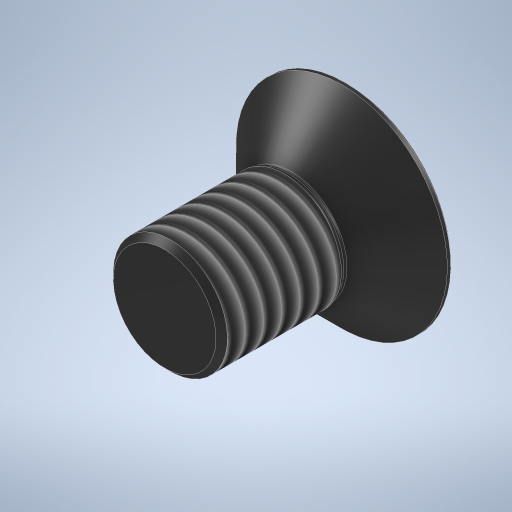
# Autodesk Inventor part: FSCM5x8
Saved by Autodesk Inventor 2024 (Build 280153000, 153)
## iProperties
Created: 2024-09-05
Part Number: FSCM5x8
Material: Stainless Steel
Document SubType Name: Modeling
Designer: Ishaan
Density: 8 g/cm^3
Appearance: Iron Gray
Author: Ishaan
Autodesk Inventor part; units mm, degrees
ref_plane "YZ Plane" through (0, 0, 0) normal (1, 0, 0) x (0, 1, 0)
ref_plane "XZ Plane" through (0, 0, 0) normal (0, 1, 0) x (-1, 0, 0)
ref_plane "XY Plane" through (0, 0, 0) normal (0, 0, 1) x (1, 0, 0)
sketch "Sketch3" plane through (0, 0, 0) normal (1, 0, 0) x (0, 1, 0)
  line L0 (0, 0) -> (0, 8)
  line L1 (0, 8) -> (2.5, 8)
  line L2 (2.5, 8) -> (2.5, 2.6578)
  line L3 (2.5, 2.6578) -> (2.4293, 2.5871)
  line L4 (4.625, 0) -> (0, 0)
  line L5 (2.4293, 2.4457) -> (4.625, 0.25)
  line L6 (4.625, 0.25) -> (4.625, 0)
  arc A0 (2.4293, 2.5871) -> (2.4293, 2.4457) centre (2.5, 2.5164) ccw
  dimension "d37" = 4.625
  dimension "d38" = 2.5
  dimension "d39" = 8
  dimension "d40" = 0.25
  dimension "d41" = 45
  dimension "d42" = 0.1
  constraints: 14 end point, 3 perpendicular, 2 point on circle, 2 tangent, 2 vertical, 1 centre point, 1 parallel, 1 point on line
  measures "d37" distance from line of L0 L4.start
  measures "d38" distance between parallel lines of L0 L2
  measures "d39" distance between parallel lines of L4 L1
  measures "d40" distance of L5.end L4.start
  measures "d41" angle of L5 L4
  measures "d42" radius of A0
revolve "Revolution1" add sketch "Sketch3" angle 360 about axis through (0, 0, 0) along (0, 0, 1)
fillet "Fillet1" radius 0.25 1 edges at (0, -2.5, 2.6578)
thread "Thread1" size "M5x0.8" class "6g" standard "ANSI Metric M Profile" full length
chamfer "Chamfer1" distance 0.1 angle 45 1 edges at (0, -4.625, 0)
sketch "Sketch2" plane through (0, 0, 0) normal (0, 0, 1) x (1, 0, 0)
  circle A0 centre (0, 0) radius 1.97 construction
  line L0 (1.64, 0) -> (0.82, -1.4203) construction
  line L1 (0.82, -1.4203) -> (-0.82, -1.4203) construction
  line L2 (-0.82, -1.4203) -> (-1.64, 0) construction
  line L3 (-1.64, 0) -> (-0.82, 1.4203) construction
  line L4 (-0.82, 1.4203) -> (0.82, 1.4203) construction
  line L5 (0.82, 1.4203) -> (1.64, 0) construction
  circle A1 centre (1.64, 0) radius 0.33
  circle A2 centre (0.82, -1.4203) radius 0.33
  circle A3 centre (-0.82, -1.4203) radius 0.33
  circle A4 centre (-1.64, 0) radius 0.33
  circle A5 centre (-0.82, 1.4203) radius 0.33
  circle A6 centre (0.82, 1.4203) radius 0.33
  circle A7 centre (1.9406, 1.1204) radius 0.83
  circle A8 centre (1.9406, -1.1204) radius 0.83
  circle A9 centre (0, -2.2408) radius 0.83
  circle A10 centre (-1.9406, -1.1204) radius 0.83
  circle A11 centre (-1.9406, 1.1204) radius 0.83
  circle A12 centre (0, 2.2408) radius 0.83
  circle A13 centre (0, 0) radius 1.25
  point P0 (-0.5867, 1.6537)
  point P1 (-1.1388, 1.335)
  point P2 (-1.7255, 0.3187)
  point P3 (-1.7255, -0.3187)
  point P4 (-1.1388, -1.335)
  point P5 (-0.5867, -1.6537)
  point P6 (0.5867, -1.6537)
  point P7 (1.1388, -1.335)
  point P8 (1.7255, -0.3187)
  point P9 (1.7255, 0.3187)
  point P10 (1.1388, 1.335)
  point P11 (0.5867, 1.6537)
  dimension "d30" = 3.94
  dimension "d31" = 0.66
  dimension "d32" = 1.66
  dimension "d33" = 2.5
  constraints: 14 centre point, 13 tangent, 12 end point, 10 equal radius, 9 coincident, 1 horizontal, 13 other
  measures "d30" diameter of A0
  measures "d31" diameter of A1
  measures "d32" diameter of A7
  measures "d33" diameter of A13
hole "Hole1" at (0, 0, 0) direction (0, 0, 1) diameter 2.5 depth 2.5 tip angle 150
chamfer "Chamfer2" distance 0.5 distance2 0.8 1 edges at (0, -1.25, 0) measured on face at (0, -1.25, 0.5)
extrude "Extrusion4" cut sketch "Sketch2" along normal up to surface contours A1 | A1 A8 A2 A9 A3 A10 A4 A11 A5 A12 A6 A7 | A6 | A2 | A5 | A3 | A4 | A13 round surface about axis through (0, 0, 2.6675) along (0, 0, 1) radius 0.625 half angle -75 far side no
chamfer "Chamfer3" distance 0.25 angle 45 1 edges at (0, -2.5, 8)
equation "\"d23\" = d33"
body "Solid1"
body "Solid2"
